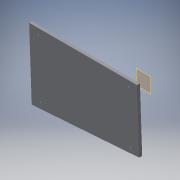
# Autodesk Inventor part: Skirt
Saved by Autodesk Inventor 2019.2 (Build 232265000, 265)
## iProperties
Created: 2018-11-10
Part Number: Skirt
Material: Generic
Document SubType Name: Modeling
Designer: eroldan
Density: 1 g/cm^3
Appearance: Default
Author: eroldan
Autodesk Inventor part; units mm, degrees
ref_plane "YZ Plane" through (0, 0, 0) normal (1, 0, 0) x (0, 1, 0)
ref_plane "XZ Plane" through (0, 0, 0) normal (0, 1, 0) x (-1, 0, 0)
ref_plane "Work Plane1" through (0, 0, 20.6375) normal (0, 0, 1) x (1, 0, 0)
sketch "Sketch2" plane through (0, 0, 20.6375) normal (0, 0, 1) x (1, 0, 0)
  line L0 (-10.7157, -11.1125) -> (-145.5988, -11.1125)
  line L1 (-142.6045, -93.4325) -> (-8.0778, -83.6332)
  line L2 (-10.7157, -11.1125) -> (-8.0778, -83.6332)
  line L3 (-145.5988, -11.1125) -> (-142.6045, -93.4325)
  line L4 (-1.8511, -89.2153) -> (-148.3933, -99.8899)
  line L5 (-148.3933, -99.8899) -> (-151.8414, -5.0928)
  line L6 (-151.8414, -5.0928) -> (-4.9109, -5.0928)
  line L7 (-4.9109, -5.0928) -> (-1.8511, -89.2153)
  point P0 (0, 0)
  constraints: 16 end point, 2 parallel, 1 horizontal, 8 other
extrude "Extrusion1" add sketch "Sketch2" along normal blind 4 contours L2 L1 L3 L0 | L4 L5 L6 L7
sketch "Sketch3" plane through (0, 0, 24.6375) normal (0, 0, 1) x (1, 0, 0)
  line L0 (-151.8414, -5.0928) -> (-148.3933, -99.8899) projected
  line L1 (-1.8511, -89.2153) -> (-4.9109, -5.0928) projected
  line L2 (-3.381, -47.1541) -> (-150.1174, -52.4913) construction
  point P0 (0, 0)
  point P1 (-16.4055, -12.6992)
  point P2 (-139.9086, -13.2096)
  point P3 (-13.8679, -82.4641)
  point P4 (-137.0817, -90.9276)
  constraints: 2 end point, 2 midpoint, 2 symmetric about line
hole "Hole1" at (-16.4055, -12.6992, 24.6375) at (-139.9086, -13.2096, 24.6375) at (-13.8679, -82.4641, 24.6375) at (-137.0817, -90.9276, 24.6375) direction (0, 0, -1) diameter 2 end through all
body "Solid1"
